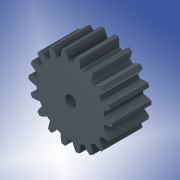
# Autodesk Inventor part: BA006
Saved by Autodesk Inventor 2017 SP1 (Build 210196100, 196)
## iProperties
Created: 2017-06-15
Part Number: BA006
Material: ABS Plastic
Document SubType Name: Modeling
Designer: zallen
Density: 1.06 g/cm^3
Appearance: CR Dark Blue
Author: zallen
Autodesk Inventor part; units mm, degrees
ref_plane "YZ Plane" through (0, 0, 0) normal (1, 0, 0) x (0, 1, 0)
ref_plane "XZ Plane" through (0, 0, 0) normal (0, 1, 0) x (-1, 0, 0)
ref_plane "XY Plane" through (0, 0, 0) normal (0, 0, 1) x (1, 0, 0)
sketch "Sketch1" plane through (0, 0, 0) normal (0, 0, 1) x (1, 0, 0)
  circle A0 centre (0, 0) radius 17.5
  arc A1 (21.3853, 0.9) -> (17.3853, 2) centre (15.4462, -12.8741) ccw
  arc A2 (17.3853, -2) -> (21.3853, -0.9) centre (15.4462, 12.8741) ccw
  arc A3 (21.3853, -0.9) -> (21.3853, 0.9) centre (1.4056, 0) ccw
  line L0 (0, 0) -> (21.7354, 0) construction
  arc A4 (17.3853, -2) -> (17.3853, 2) centre (0, 0) ccw
  arc A5 (19.7878, 8.1599) -> (15.6528, 7.8255) centre (18.9179, -6.8148) ccw
  arc A6 (20.4035, 6.4685) -> (19.7878, 8.1599) centre (1.3208, 0.4807) ccw
  arc A7 (17.0209, 4.0668) -> (20.4035, 6.4685) centre (10.1115, 17.3806) ccw
  circle A8 centre (0, 0) radius 17.5
  arc A9 (17.0209, 4.0668) -> (15.6528, 7.8255) centre (0, 0) ccw
  arc A10 (15.8036, 14.4357) -> (12.0324, 12.7072) centre (20.1078, 0.0665) ccw
  arc A11 (16.9606, 13.0568) -> (15.8036, 14.4357) centre (1.0768, 0.9035) ccw
  arc A12 (14.6035, 9.643) -> (16.9606, 13.0568) centre (3.5571, 19.7908) ccw
  circle A13 centre (0, 0) radius 17.5
  arc A14 (14.6035, 9.643) -> (12.0324, 12.7072) centre (0, 0) ccw
  arc A15 (9.9132, 18.9702) -> (6.9606, 16.0561) centre (18.8724, 6.9397) ccw
  arc A16 (11.4721, 18.0702) -> (9.9132, 18.9702) centre (0.7028, 1.2173) ccw
  arc A17 (10.4247, 14.0561) -> (11.4721, 18.0702) centre (-3.4262, 19.8139) ccw
  circle A18 centre (0, 0) radius 17.5
  arc A19 (10.4247, 14.0561) -> (6.9606, 16.0561) centre (0, 0) ccw
  arc A20 (2.8272, 21.2167) -> (1.0493, 17.4685) centre (15.3607, 12.976) ccw
  arc A21 (4.5999, 20.9042) -> (2.8272, 21.2167) centre (0.2441, 1.3842) ccw
  arc A22 (4.9885, 16.7739) -> (4.5999, 20.9042) centre (-9.9963, 17.4471) ccw
  circle A23 centre (0, 0) radius 17.5
  arc A24 (4.9885, 16.7739) -> (1.0493, 17.4685) centre (0, 0) ccw
  arc A25 (-4.5999, 20.9042) -> (-4.9885, 16.7739) centre (9.9963, 17.4471) ccw
  arc A26 (-2.8272, 21.2167) -> (-4.5999, 20.9042) centre (-0.2441, 1.3842) ccw
  arc A27 (-1.0493, 17.4685) -> (-2.8272, 21.2167) centre (-15.3607, 12.976) ccw
  circle A28 centre (0, 0) radius 17.5
  arc A29 (-1.0493, 17.4685) -> (-4.9885, 16.7739) centre (0, 0) ccw
  arc A30 (-11.4721, 18.0702) -> (-10.4247, 14.0561) centre (3.4262, 19.8139) ccw
  arc A31 (-9.9132, 18.9702) -> (-11.4721, 18.0702) centre (-0.7028, 1.2173) ccw
  arc A32 (-6.9606, 16.0561) -> (-9.9132, 18.9702) centre (-18.8724, 6.9397) ccw
  circle A33 centre (0, 0) radius 17.5
  arc A34 (-6.9606, 16.0561) -> (-10.4247, 14.0561) centre (0, 0) ccw
  arc A35 (-16.9606, 13.0568) -> (-14.6035, 9.643) centre (-3.5571, 19.7908) ccw
  arc A36 (-15.8036, 14.4357) -> (-16.9606, 13.0568) centre (-1.0768, 0.9035) ccw
  arc A37 (-12.0324, 12.7072) -> (-15.8036, 14.4357) centre (-20.1078, 0.0665) ccw
  circle A38 centre (0, 0) radius 17.5
  arc A39 (-12.0324, 12.7072) -> (-14.6035, 9.643) centre (0, 0) ccw
  arc A40 (-20.4035, 6.4685) -> (-17.0209, 4.0668) centre (-10.1115, 17.3806) ccw
  arc A41 (-19.7878, 8.1599) -> (-20.4035, 6.4685) centre (-1.3208, 0.4807) ccw
  arc A42 (-15.6528, 7.8255) -> (-19.7878, 8.1599) centre (-18.9179, -6.8148) ccw
  circle A43 centre (0, 0) radius 17.5
  arc A44 (-15.6528, 7.8255) -> (-17.0209, 4.0668) centre (0, 0) ccw
  arc A45 (-21.3853, -0.9) -> (-17.3853, -2) centre (-15.4462, 12.8741) ccw
  arc A46 (-21.3853, 0.9) -> (-21.3853, -0.9) centre (-1.4056, 0) ccw
  arc A47 (-17.3853, 2) -> (-21.3853, 0.9) centre (-15.4462, -12.8741) ccw
  circle A48 centre (0, 0) radius 17.5
  arc A49 (-17.3853, 2) -> (-17.3853, -2) centre (0, 0) ccw
  arc A50 (-19.7878, -8.1599) -> (-15.6528, -7.8255) centre (-18.9179, 6.8148) ccw
  arc A51 (-20.4035, -6.4685) -> (-19.7878, -8.1599) centre (-1.3208, -0.4807) ccw
  arc A52 (-17.0209, -4.0668) -> (-20.4035, -6.4685) centre (-10.1115, -17.3806) ccw
  circle A53 centre (0, 0) radius 17.5
  arc A54 (-17.0209, -4.0668) -> (-15.6528, -7.8255) centre (0, 0) ccw
  arc A55 (-15.8036, -14.4357) -> (-12.0324, -12.7072) centre (-20.1078, -0.0665) ccw
  arc A56 (-16.9606, -13.0568) -> (-15.8036, -14.4357) centre (-1.0768, -0.9035) ccw
  arc A57 (-14.6035, -9.643) -> (-16.9606, -13.0568) centre (-3.5571, -19.7908) ccw
  circle A58 centre (0, 0) radius 17.5
  arc A59 (-14.6035, -9.643) -> (-12.0324, -12.7072) centre (0, 0) ccw
  arc A60 (-9.9132, -18.9702) -> (-6.9606, -16.0561) centre (-18.8724, -6.9397) ccw
  arc A61 (-11.4721, -18.0702) -> (-9.9132, -18.9702) centre (-0.7028, -1.2173) ccw
  arc A62 (-10.4247, -14.0561) -> (-11.4721, -18.0702) centre (3.4262, -19.8139) ccw
  circle A63 centre (0, 0) radius 17.5
  arc A64 (-10.4247, -14.0561) -> (-6.9606, -16.0561) centre (0, 0) ccw
  arc A65 (-2.8272, -21.2167) -> (-1.0493, -17.4685) centre (-15.3607, -12.976) ccw
  arc A66 (-4.5999, -20.9042) -> (-2.8272, -21.2167) centre (-0.2441, -1.3842) ccw
  arc A67 (-4.9885, -16.7739) -> (-4.5999, -20.9042) centre (9.9963, -17.4471) ccw
  circle A68 centre (0, 0) radius 17.5
  arc A69 (-4.9885, -16.7739) -> (-1.0493, -17.4685) centre (0, 0) ccw
  arc A70 (4.5999, -20.9042) -> (4.9885, -16.7739) centre (-9.9963, -17.4471) ccw
  arc A71 (2.8272, -21.2167) -> (4.5999, -20.9042) centre (0.2441, -1.3842) ccw
  arc A72 (1.0493, -17.4685) -> (2.8272, -21.2167) centre (15.3607, -12.976) ccw
  circle A73 centre (0, 0) radius 17.5
  arc A74 (1.0493, -17.4685) -> (4.9885, -16.7739) centre (0, 0) ccw
  arc A75 (11.4721, -18.0702) -> (10.4247, -14.0561) centre (-3.4262, -19.8139) ccw
  arc A76 (9.9132, -18.9702) -> (11.4721, -18.0702) centre (0.7028, -1.2173) ccw
  arc A77 (6.9606, -16.0561) -> (9.9132, -18.9702) centre (18.8724, -6.9397) ccw
  circle A78 centre (0, 0) radius 17.5
  arc A79 (6.9606, -16.0561) -> (10.4247, -14.0561) centre (0, 0) ccw
  arc A80 (16.9606, -13.0568) -> (14.6035, -9.643) centre (3.5571, -19.7908) ccw
  arc A81 (15.8036, -14.4357) -> (16.9606, -13.0568) centre (1.0768, -0.9035) ccw
  arc A82 (12.0324, -12.7072) -> (15.8036, -14.4357) centre (20.1078, -0.0665) ccw
  circle A83 centre (0, 0) radius 17.5
  arc A84 (12.0324, -12.7072) -> (14.6035, -9.643) centre (0, 0) ccw
  arc A85 (20.4035, -6.4685) -> (17.0209, -4.0668) centre (10.1115, -17.3806) ccw
  arc A86 (19.7878, -8.1599) -> (20.4035, -6.4685) centre (1.3208, -0.4807) ccw
  arc A87 (15.6528, -7.8255) -> (19.7878, -8.1599) centre (18.9179, 6.8148) ccw
  circle A88 centre (0, 0) radius 17.5
  arc A89 (15.6528, -7.8255) -> (17.0209, -4.0668) centre (0, 0) ccw
  dimension "d0" = 35
  dimension "d3" = 15
  dimension "d4" = 15
  dimension "d5" = 4
  dimension "d6" = 20
  dimension "d7" = 1.8
  dimension "d10" = 360
  dimension "d20" = 2
  constraints: 180 point on circle, 90 centre point, 2 end point, 2 symmetric about line, 2 vertical alignment, 1 coincident, 1 concentric, 1 horizontal, 253 other
  measures "d0" diameter of A0
  measures "d3" radius of A1
  measures "d4" radius of A2
  measures "d5" horizontal distance of A1.start A0.start
  measures "d6" radius of A3
  measures "d7" distance of A2.end A1.start
  measures "d20" distance from line of L0 A0.start
extrude "Extrusion1" add sketch "Sketch1" along normal blind 20
sketch "Sketch2" plane through (0, 0, 20) normal (0, 0, 1) x (1, 0, 0)
  circle A0 centre (0, 0) radius 2.75
  dimension "d14" = 5.5
  constraints: 1 centre point, 1 coincident
  measures "d14" diameter of A0
extrude "Extrusion2" cut sketch "Sketch2" against normal through all
body "Solid1"
